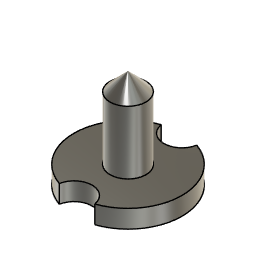
مسمار v3 (Autodesk Fusion 360 design; units mm, degrees)
Autodesk Fusion 360 part; units mm, degrees
sketch "Sketch1" plane through (0, 0, 0) normal (1, 0, 0) x (0, 1, 0)
  line L0 (0, 0) -> (0, 40)
  line L1 (0, 40) -> (20, 20)
  line L2 (38.614, 36.3802) -> (38.614, 30)
  line L3 (20, 20) -> (20, 0)
  line L4 (20, 0) -> (20, -50)
  line L5 (20, -50) -> (60, -50)
  line L6 (60, -50) -> (60, -70)
  line L7 (60, -70) -> (0, -70)
  line L8 (0, -70) -> (0, 40)
  constraint coincident L0.start origin
  constraint vertical L0
  constraint parallel L0 L3
  constraint parallel L3 L4
  constraint perpendicular L4 L5
  constraint perpendicular L5 L6
  constraint perpendicular L6 L7
  constraint perpendicular L7 L8
revolve "Revolve1" add sketch "Sketch1" angle 360 about axis through (0, 0, 1.75) along (0, 0, 1)
sketch "Sketch2" plane through (0, 0, 0) normal (1, 0, 0) x (0, 1, 0)
  line L0 (60, -50) -> (40, -50)
  line L1 (40, -50) -> (40, -70)
  line L2 (40, -70) -> (60, -70)
  line L3 (60, -70) -> (60, -50)
  constraint horizontal L0
  constraint vertical L1
  constraint horizontal L2
  constraint vertical L3
revolve "Revolve2" cut sketch "Sketch2" angle 360 about axis through (0, 60, -70) along (0, 0, 1)
mirror "Mirror1" about plane through (0, 0, 0) normal (0, 1, 0) of "Revolve2"
